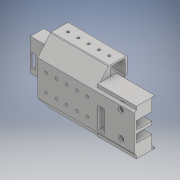
# Autodesk Inventor part: MagnetHousing_SmallGrad
Saved by Autodesk Inventor 2017 (Build 210142000, 142)
## iProperties
Created: 2017-04-05
Part Number: MagnetHousing_SmallGrad
Material: Generic
Document SubType Name: Modeling
Designer: greer_000
Density: 1 g/cm^3
Appearance: Default
Mass: 46.9919 g
Surface Area: 340.055 cm^2
Volume: 46.9919 cm^3
Author: greer_000
Autodesk Inventor part; units mm, degrees
ref_plane "YZ Plane" through (0, 0, 0) normal (1, 0, 0) x (0, 1, 0)
ref_plane "XZ Plane" through (0, 0, 0) normal (0, 1, 0) x (-1, 0, 0)
ref_plane "XY Plane" through (0, 0, 0) normal (0, 0, 1) x (1, 0, 0)
sketch "Sketch1" plane through (0, 0, 0) normal (1, 0, 0) x (0, 1, 0)
  line L0 (0, 0) -> (0, 17)
  line L1 (0, 17) -> (12.3002, 31.677)
  line L2 (13.0667, 32.0347) -> (29.3, 32.0347)
  line L3 (30.3, 31.0347) -> (30.3, 16.2862)
  line L4 (16.75, 10.8595) -> (16.75, 0)
  line L5 (29.5781, 15.3257) -> (17.4719, 11.8201)
  line L6 (0, 0) -> (0, -17)
  line L7 (0, -17) -> (12.3002, -31.677)
  line L8 (13.0667, -32.0347) -> (29.3, -32.0347)
  line L9 (30.3, -31.0347) -> (30.3, -16.2862)
  line L10 (16.75, -10.8595) -> (16.75, 0)
  line L11 (29.5781, -15.3257) -> (17.4719, -11.8201)
  arc A0 (29.3, -32.0347) -> (30.3, -31.0347) centre (29.3, -31.0347) ccw
  arc A1 (30.3, -16.2862) -> (29.5781, -15.3257) centre (29.3, -16.2862) ccw
  arc A2 (29.5781, 15.3257) -> (30.3, 16.2862) centre (29.3, 16.2862) ccw
  arc A3 (30.3, 31.0347) -> (29.3, 32.0347) centre (29.3, 31.0347) ccw
  arc A4 (13.0667, 32.0347) -> (12.3002, 31.677) centre (13.0667, 31.0347) ccw
  arc A5 (12.3002, -31.677) -> (13.0667, -32.0347) centre (13.0667, -31.0347) ccw
  line L12 (17.4719, 11.8201) -> (16.75, 11.6111)
  line L13 (16.75, 11.6111) -> (16.75, 10.8595)
  line L14 (17.4719, -11.8201) -> (16.75, -11.611)
  line L15 (16.75, -11.611) -> (16.75, -10.8595)
  point P0 (12.6, 32.0347)
  point P1 (30.3, 32.0347)
  point P2 (30.3, 15.5347)
  point P3 (12.6, -32.0347)
  point P4 (30.3, -32.0347)
  point P5 (30.3, -15.5347)
  point P6 (16.75, -11.6111)
  dimension "d1" = 17
  dimension "d3" = 17.7
  dimension "d4" = 30.3
  dimension "d5" = 16.5
  dimension "d6" = 16.75
  dimension "d7" = 11.6111
  dimension "d186" = 11.6111
  dimension "d187" = 17.7
  dimension "d188" = 30.3
  dimension "d189" = 16.5
  dimension "d191" = 15.0347
  dimension "d192" = 17
  dimension "d297" = 15.0347
  dimension "d308" = 3.9236
  dimension "d309" = 3.9236
  dimension "d325" = 1
  constraints: 32 end point, 16 point on line, 12 point on circle, 12 tangent, 6 centre point, 5 equal radius, 5 vertical, 1 horizontal
  measures "d1" distance of L0.start L0.end
  measures "d3" distance of point (12.6, 32.035) point (30.3, 32.035)
  measures "d4" horizontal distance of L0.end point (30.3, 32.035)
  measures "d5" distance of point (30.3, 32.035) point (30.3, 15.535)
  measures "d6" distance between parallel lines of L4 L0
  measures "d7" distance of L12.end L4.end
  measures "d186" distance of point (16.75, -11.611) L4.end
  measures "d187" distance of point (12.6, -32.035) point (30.3, -32.035)
  measures "d188" distance from line of L7.start L9
  measures "d189" distance of point (30.3, -32.035) point (30.3, -15.535)
  measures "d191" vertical distance of point (12.6, -32.035) L7.start
  measures "d192" distance of L0.start L7.start
  measures "d297" vertical distance of point (12.6, 32.035) L0.end
  measures "d308" vertical distance of L12.end point (30.3, 15.535)
  measures "d309" vertical distance of point (30.3, -15.535) point (16.75, -11.611)
  measures "d325" radius of A0
extrude "Extrusion1" add sketch "Sketch1" against normal blind 56.3
sketch "Sketch2" plane through (0, 0, 0) normal (1, 0, 0) x (0, 0, -1)
  line L0 (-29.4847, 28.55) -> (-16.5847, 28.55)
  line L1 (-15.5847, 27.55) -> (-15.5847, 14.325)
  line L2 (-30.4847, 15.325) -> (-30.4847, 27.55)
  line L3 (-32.0347, 13.0667) -> (-32.0347, 29.3) projected
  line L4 (17, 0) -> (-17, 0) projected
  line L5 (-11.6111, 16.75) -> (11.6111, 16.75) projected
  line L6 (0, 16.75) -> (0, 3.3802)
  line L7 (29.4847, 28.55) -> (16.5847, 28.55)
  line L8 (15.5847, 27.55) -> (15.5847, 14.325)
  line L9 (15.5847, 14.325) -> (29.4847, 14.325)
  line L10 (30.4847, 15.325) -> (30.4847, 27.55)
  line L11 (-14.4375, 15.9) -> (14.438, 15.9)
  line L12 (14.438, 15.9) -> (14.438, 1.75)
  line L13 (14.438, 1.75) -> (-14.4375, 1.75)
  line L14 (-14.4375, 1.75) -> (-14.4375, 15.9)
  line L15 (-31.0347, 30.3) -> (-16.2862, 30.3) projected
  arc A0 (-15.5847, 27.55) -> (-16.5847, 28.55) centre (-16.5847, 27.55) ccw
  arc A1 (-29.4847, 28.55) -> (-30.4847, 27.55) centre (-29.4847, 27.55) ccw
  arc A2 (16.5847, 28.55) -> (15.5847, 27.55) centre (16.5847, 27.55) ccw
  arc A3 (30.4847, 27.55) -> (29.4847, 28.55) centre (29.4847, 27.55) ccw
  arc A4 (29.4847, 14.325) -> (30.4847, 15.325) centre (29.4847, 15.325) ccw
  line L16 (-15.5847, 14.325) -> (-29.4847, 14.325)
  line L17 (-30.4847, 15.325) -> (-30.4847, 15.325)
  arc A5 (-30.4847, 15.325) -> (-29.4847, 14.325) centre (-29.4847, 15.325) ccw
  line L18 (-16.0847, 14.325) -> (-28.7847, 14.325) construction
  line L19 (-28.7847, 14.325) -> (-28.7847, 27.025) construction
  line L20 (-28.7847, 27.025) -> (-16.0847, 27.025) construction
  line L21 (-16.0847, 27.025) -> (-16.0847, 14.325) construction
  line L22 (-28.7847, 20.675) -> (-4.4905, 20.675) construction
  line L23 (-12.9889, 15.4) -> (6.9303, 15.4) construction
  line L24 (16.0847, 14.325) -> (28.7847, 14.325) construction
  line L25 (28.7847, 14.325) -> (28.7847, 27.025) construction
  line L26 (28.7847, 27.025) -> (16.0847, 27.025) construction
  line L27 (16.0847, 27.025) -> (16.0847, 14.325) construction
  line L28 (16.0847, 20.675) -> (4.3729, 20.675) construction
  line L29 (-22.4347, 27.025) -> (-22.4347, 13.0667) construction
  point P0 (0, 0)
  point P1 (-30.4847, 28.55)
  point P2 (-15.5847, 28.55)
  point P3 (-30.4847, 14.325)
  point P4 (-32.0347, 12.6)
  point P5 (-32.0347, 30.3)
  point P6 (30.4847, 28.55)
  point P7 (15.5847, 28.55)
  point P8 (30.4847, 14.325)
  point P9 (-15.5347, 30.3)
  point P10 (-10.8595, 16.75)
  point P11 (10.8595, 16.75)
  dimension "d11" = 1.55
  dimension "d15" = 1.75
  dimension "d16" = 14.4375
  dimension "d17" = 14.438
  dimension "d295" = 1.75
  dimension "d296" = 0.85
  dimension "d316" = 15.5847
  dimension "d320" = 1
  dimension "d324" = 1
  dimension "d397" = 12.225
  dimension "d399" = 13.225
  dimension "d400" = 12.225
  dimension "d406" = 1
  dimension "d407" = 12.7
  dimension "d408" = 12.7
  dimension "d409" = 0.5
  dimension "d410" = 0.5
  dimension "d411" = 12.7
  dimension "d412" = 12.7
  dimension "d413" = 0.5
  constraints: 52 end point, 16 point on line, 12 point on circle, 12 tangent, 6 centre point, 6 horizontal, 6 parallel, 4 midpoint, 4 perpendicular, 4 symmetric about line, 3 equal radius, 1 vertical
  measures "d11" distance between parallel lines of L2 L3
  measures "d15" distance between parallel lines of L13 L4
  measures "d16" distance between parallel lines of L6 L14
  measures "d17" distance between parallel lines of L6 L12
  measures "d295" distance between parallel lines of L15 L0
  measures "d296" distance between parallel lines of L5 L11
  measures "d316" distance between parallel lines of L6 L1
  measures "d320" radius of A0
  measures "d324" radius of A2
  measures "d397" distance of L2.start L2.end
  measures "d399" distance of L1.start L1.end
  measures "d400" distance of L10.start L10.end
  measures "d406" radius of A5
  measures "d407" distance of L19.end L20.end
  measures "d408" distance of L18.end L19.end
  measures "d409" distance between parallel lines of L1 L21
  measures "d410" distance between parallel lines of L11 L23
  measures "d411" distance of L26.end L25.end
  measures "d412" distance of L25.end L24.end
  measures "d413" distance between parallel lines of L8 L27
extrude "Extrusion2" cut sketch "Sketch2" against normal up to next
sketch "Sketch35" plane through (0, 0, 0) normal (1, 0, 0) x (0, 0, -1)
  line L0 (-11.6111, 16.75) -> (11.6111, 16.75) projected
  line L1 (-11.6111, 16.75) -> (-15.7347, 16.75)
  line L2 (-15.7347, 16.75) -> (-15.7347, 15.9)
  line L3 (-15.7347, 15.9) -> (15.5847, 15.9)
  line L4 (15.5847, 14.325) -> (15.5847, 27.55) projected
  line L5 (15.5847, 15.9) -> (15.5847, 16.75)
  line L6 (15.5847, 16.75) -> (11.6111, 16.75)
  line L7 (-11.6111, 16.75) -> (11.6111, 16.75)
  point P0 (0, 0)
  point P1 (15.5847, 28.8)
  point P2 (-10.8595, 16.75)
  point P3 (10.8595, 16.75)
  constraints: 12 end point, 2 collinear, 2 vertical, 1 horizontal, 1 perpendicular, 1 point on line
extrude "Extrusion32" add sketch "Sketch35" along normal blind 8.062
sketch "Sketch36" plane through (-56.3, 16.75, -11.611) normal (0, 1, 0) x (1, 0, 0)
  circle A0 centre (61.362, -17.6111) radius 1.505
  circle A1 centre (61.362, -11.6111) radius 1.505
  circle A2 centre (61.362, -5.6111) radius 1.505
  line L0 (64.362, 3.9736) -> (64.362, -27.3457) projected
  point P0 (56.3, -11.6111)
  dimension "d195" = 3.01
  dimension "d196" = 3.01
  dimension "d197" = 3.01
  dimension "d198" = 3
  dimension "d200" = 3
  dimension "d201" = 0
  dimension "d202" = 3
  dimension "d203" = 6
  dimension "d204" = 6
  constraints: 3 centre point
  measures "d195" diameter of A0
  measures "d196" diameter of A1
  measures "d197" diameter of A2
  measures "d198" distance from line of L0 A0.centre
  measures "d200" distance from line of L0 A2.centre
  measures "d201" vertical distance of point (56.3, -11.611) A1.centre
  measures "d202" distance from line of A1.centre L0
  measures "d203" distance of A2.centre A1.centre
  measures "d204" distance of A0.centre A1.centre
extrude "Extrusion33" cut sketch "Sketch36" against normal blind 8.062
sketch "Sketch37" plane through (0, 14.325, -15.5847) normal (0, 0, -1) x (-1, 0, 0)
  line L0 (0, 2.425) -> (-8.062, 2.425) projected
  line L1 (0, 1.575) -> (-8.062, 1.575) projected
  line L2 (-8.062, 2.425) -> (0, 2.425)
  line L3 (0, 2.425) -> (0, 1.075)
  line L4 (0, 1.075) -> (-8.062, 1.075)
  line L5 (-8.062, 1.075) -> (-8.062, 2.425)
  point P0 (0, -14.325)
  constraints: 8 end point, 2 parallel, 1 horizontal, 1 perpendicular, 1 other
extrude "Extrusion34" add sketch "Sketch37" along normal blind 4.9105
sketch "Sketch38" plane through (0, 14.325, 15.5847) normal (0, 0, 1) x (1, 0, 0)
  line L0 (8.062, 2.425) -> (8.062, 1.575) projected
  line L1 (8.062, 2.425) -> (0, 2.425)
  line L2 (0, 2.425) -> (0, 1.575)
  line L3 (0, 1.575) -> (8.062, 1.575)
  line L4 (8.062, 1.575) -> (8.062, 2.425)
  point P0 (0, -14.325)
  constraints: 8 end point, 2 parallel, 1 horizontal, 1 perpendicular
extrude "Extrusion35" add sketch "Sketch38" along normal blind 4.9105
sketch "Sketch39" plane through (8.062, 0, 0) normal (1, 0, 0) x (0, 0, -1)
  line L0 (-15.5847, 16.75) -> (-20.4952, 16.75) projected
  line L1 (15.5847, 15.4) -> (20.4952, 15.4) projected
  line L2 (-20.4952, 16.75) -> (20.4952, 16.75)
  line L3 (20.4952, 16.75) -> (20.4952, 15.4)
  line L4 (20.4952, 15.4) -> (-20.4952, 15.4)
  line L5 (-20.4952, 15.4) -> (-20.4952, 16.75)
  point P0 (0, 0)
  point P1 (15.5847, 15.9)
  constraints: 8 end point, 2 parallel, 1 horizontal, 1 perpendicular, 1 other
extrude "Extrusion36" add sketch "Sketch39" along normal blind 29.6
sketch "Sketch40" plane through (-56.3, 16.75, -11.611) normal (0, 1, 0) x (1, 0, 0)
  line L0 (85.241, 1.9681) -> (91.351, 1.9681)
  line L1 (91.351, 1.9681) -> (91.351, 7.4181)
  line L2 (91.351, 7.4181) -> (85.241, 7.4181)
  line L3 (85.241, 7.4181) -> (85.241, 1.9681)
  line L4 (56.3, 8.8841) -> (93.962, 8.8841) projected
  line L5 (93.962, -32.1062) -> (93.962, 8.8841) projected
  circle A0 centre (80.723, -1.2209) radius 6.25
  point P0 (56.3, -11.6111)
  dimension "d213" = 6.11
  dimension "d214" = 5.45
  dimension "d215" = 1.466
  dimension "d216" = 2.611
  dimension "d217" = 12.5
  dimension "d218" = 10.105
  dimension "d219" = 13.239
  constraints: 8 end point, 2 parallel, 1 centre point, 1 horizontal, 1 perpendicular
  measures "d213" distance of L1.end L2.end
  measures "d214" distance of L2.end L0.start
  measures "d215" distance between parallel lines of L4 L2
  measures "d216" distance between parallel lines of L5 L1
  measures "d217" diameter of A0
  measures "d218" distance from line of L4 A0.centre
  measures "d219" distance from line of L5 A0.centre
extrude "Extrusion37" cut sketch "Sketch40" against normal blind 29.6
sketch "Sketch41" plane through (-56.3, 16.75, -11.611) normal (0, 1, 0) x (1, 0, 0)
  line L0 (84.662, -21.7659) -> (93.962, -21.7659)
  line L1 (93.962, -21.7659) -> (93.962, -13.7659)
  line L2 (93.962, -13.7659) -> (84.662, -13.7659)
  line L3 (84.662, -13.7659) -> (84.662, -21.7659)
  line L4 (84.662, -10.8659) -> (93.962, -10.8659)
  line L5 (93.962, -10.8659) -> (93.962, -2.8659)
  line L6 (93.962, -2.8659) -> (84.662, -2.8659)
  line L7 (84.662, -2.8659) -> (84.662, -10.8659)
  line L8 (56.3, 8.8841) -> (93.962, 8.8841) projected
  line L9 (93.962, 8.8841) -> (93.962, -32.1062) projected
  point P0 (56.3, -11.6111)
  dimension "d222" = 9.3
  dimension "d223" = 8
  dimension "d224" = 8
  dimension "d225" = 11.75
  dimension "d227" = 22.65
  dimension "d243" = 0
  constraints: 16 end point, 4 parallel, 2 horizontal, 2 perpendicular, 2 point on line
  measures "d222" distance of L0.start L0.end
  measures "d223" distance of L2.end L0.start
  measures "d224" distance of L6.end L4.start
  measures "d225" distance between parallel lines of L8 L6
  measures "d227" distance between parallel lines of L8 L2
  measures "d243" distance between parallel lines of L9 L1
extrude "Extrusion38" cut sketch "Sketch41" against normal blind 29.6
sketch "Sketch42" plane through (-56.3, 16.75, -11.611) normal (0, 1, 0) x (1, 0, 0)
  circle A0 centre (80.604, -25.0282) radius 6.25
  line L0 (56.3, -32.1062) -> (93.962, -32.1062) projected
  line L1 (93.962, 8.8841) -> (93.962, -32.1062) projected
  line L2 (75.873, -15.0931) -> (83.551, -15.0931)
  line L3 (83.551, -15.0931) -> (83.551, -9.6387)
  line L4 (83.551, -9.6387) -> (75.873, -9.6387)
  line L5 (75.873, -9.6387) -> (75.873, -15.0931)
  line L6 (56.3, 8.8841) -> (93.962, 8.8841) projected
  point P0 (56.3, -11.6111)
  dimension "d230" = 12.5
  dimension "d231" = 7.078
  dimension "d232" = 13.358
  dimension "d237" = 18.5228
  dimension "d238" = 5.4544
  dimension "d239" = 10.411
  dimension "d240" = 7.678
  constraints: 8 end point, 2 parallel, 1 centre point, 1 horizontal, 1 perpendicular
  measures "d230" diameter of A0
  measures "d231" distance from line of L0 A0.centre
  measures "d232" distance from line of L1 A0.centre
  measures "d237" distance between parallel lines of L6 L4
  measures "d238" distance of L4.end L2.start
  measures "d239" distance between parallel lines of L1 L3
  measures "d240" distance of L2.start L2.end
extrude "Extrusion39" cut sketch "Sketch42" against normal blind 29.6
sketch "Sketch43" plane through (-56.3, 16.75, -11.611) normal (0, 1, 0) x (1, 0, 0)
  line L0 (69.359, -17.8987) -> (73.747, -17.8987)
  line L1 (73.747, -17.8987) -> (73.747, -8.4307)
  line L2 (73.747, -8.4307) -> (69.359, -8.4307)
  line L3 (69.359, -8.4307) -> (69.359, -17.8987)
  line L4 (93.962, -21.7659) -> (93.962, -32.1062) projected
  line L5 (56.3, 8.8841) -> (93.962, 8.8841) projected
  point P0 (56.3, -11.6111)
  dimension "d244" = 9.468
  dimension "d245" = 4.388
  dimension "d246" = 20.215
  dimension "d247" = 17.3148
  constraints: 8 end point, 2 parallel, 1 horizontal, 1 perpendicular
  measures "d244" distance of L2.end L0.start
  measures "d245" distance of L1.end L2.end
  measures "d246" distance between parallel lines of L4 L1
  measures "d247" distance between parallel lines of L5 L2
extrude "Extrusion40" cut sketch "Sketch43" against normal blind 29.6
sketch "Sketch44" plane through (0, 0, 0) normal (1, 0, 0) x (0, 0, -1)
  line L0 (-14.4375, 1.75) -> (14.438, 1.75) projected
  line L1 (17, 0) -> (-17, 0) projected
  line L2 (-17, 0) -> (17, 0)
  line L3 (14.438, 1.75) -> (-14.4375, 1.75)
  line L4 (31.677, 12.3002) -> (17, 0) projected
  line L5 (14.438, 1.75) -> (19.0882, 1.75)
  line L6 (17, 0) -> (19.0882, 1.75)
  line L7 (-14.4375, 1.75) -> (-19.0882, 1.75)
  line L8 (-17, 0) -> (-31.677, 12.3002) projected
  line L9 (-19.0882, 1.75) -> (-17, 0)
  point P0 (0, 0)
  point P1 (32.0347, 12.6)
  dimension "d336" = 4.6506
  constraints: 12 end point, 3 horizontal, 2 collinear, 1 point on line
  measures "d336" distance of L0.start L7.end
extrude "Extrusion41" add sketch "Sketch44" along normal blind 37.662
sketch "Sketch45" plane through (-56.3, 16.75, -11.611) normal (0, 1, 0) x (1, 0, 0)
  line L0 (93.962, -21.7659) -> (85.935, -21.7659) projected
  line L1 (93.962, -32.1062) -> (93.962, -21.7659)
  line L2 (93.962, -21.7659) -> (85.935, -21.7659)
  arc A0 (84.662, -20.2748) -> (85.935, -21.7659) centre (80.604, -25.0282) ccw projected
  arc A1 (84.662, -29.7817) -> (85.935, -21.7659) centre (80.604, -25.0282) ccw
  line L3 (84.662, -29.7817) -> (84.662, -32.1062)
  line L4 (84.662, -32.1062) -> (93.962, -32.1062)
  line L5 (84.662, -6.0734) -> (84.662, -10.8659) projected
  line L6 (84.662, -13.7662) -> (84.662, -10.8659)
  line L7 (84.662, -10.8659) -> (93.962, -10.8659) projected
  line L8 (84.662, -10.8659) -> (93.962, -10.8659)
  line L9 (93.962, -10.8659) -> (93.962, -13.7662)
  line L10 (93.962, -28.6111) -> (93.962, 5.3889) projected
  line L11 (84.662, -13.7662) -> (93.962, -13.7662)
  line L12 (93.962, -2.8659) -> (86.7526, -2.8659) projected
  line L13 (93.962, -2.8659) -> (86.7526, -2.8659)
  arc A2 (86.7526, -2.8659) -> (86.0982, 1.9681) centre (80.723, -1.2209) ccw projected
  arc A3 (86.7526, -2.8659) -> (86.0982, 1.9681) centre (80.9931, -1.1843) ccw
  line L14 (86.0982, 1.9681) -> (91.351, 1.9681) projected
  line L15 (86.0982, 1.9681) -> (91.351, 1.9681)
  line L16 (91.351, 1.9681) -> (91.351, 7.4181)
  line L17 (91.351, 7.4181) -> (85.241, 7.4181) projected
  line L18 (91.351, 7.4181) -> (85.241, 7.4181)
  line L19 (85.241, 7.4181) -> (85.241, 8.8841)
  line L20 (56.3, 8.8841) -> (93.962, 8.8841) projected
  line L21 (93.962, 8.8841) -> (85.241, 8.8841)
  line L22 (93.962, 8.8841) -> (93.962, -2.8659)
  line L23 (56.3, -32.1062) -> (93.962, -32.1062) projected
  point P0 (56.3, -11.6111)
  point P1 (93.962, 8.0737)
  dimension "d338" = 0
  constraints: 30 end point, 5 collinear, 5 point on circle, 4 perpendicular, 3 point on line, 3 vertical, 2 centre point, 1 concentric, 1 horizontal
  measures "d338" distance between parallel lines of L23 L4
extrude "Extrusion42" add sketch "Sketch45" against normal up to surface (15 mm away) contours L1 L4 L3 A0 L0 | L6 L7 L9 L11 | L12 A3 L14 L16 L17 L19 L20 L22 L10
sketch "Sketch46" plane through (-56.3, 16.75, -11.611) normal (0, 1, 0) x (1, 0, 0)
  line L0 (56.3, -27.1957) -> (56.3, -41.0957) projected
  line L1 (84.662, -30.6992) -> (84.662, -29.7817) projected
  line L2 (56.3, -32.3892) -> (84.662, -32.3892)
  line L3 (84.662, -32.3892) -> (84.662, -29.7817)
  arc A0 (84.662, -29.7817) -> (85.935, -21.7659) centre (80.604, -25.0282) ccw projected
  arc A1 (84.662, -20.2748) -> (84.662, -29.7817) centre (80.604, -25.0282) ccw
  line L4 (84.662, -10.8659) -> (84.662, -6.0734) projected
  line L5 (84.662, -20.2748) -> (84.662, -6.0734)
  line L6 (85.241, 7.4181) -> (85.241, 3.0977) projected
  arc A2 (85.241, 3.0977) -> (84.662, -6.0734) centre (81.1316, -1.2467) ccw
  line L7 (85.241, 3.0977) -> (85.241, 7.4181)
  line L8 (85.241, 7.4181) -> (85.241, 8.8841)
  line L9 (56.3, 8.8841) -> (93.962, 8.8841) projected
  line L10 (56.3, 8.8841) -> (85.241, 8.8841)
  line L11 (56.3, 8.8841) -> (56.3, -32.3892)
  circle A3 centre (61.362, -17.6111) radius 1.505 projected
  circle A4 centre (61.362, -17.6111) radius 1.505
  circle A5 centre (61.362, -11.6111) radius 1.505 projected
  circle A6 centre (61.362, -11.6111) radius 1.505
  circle A7 centre (61.362, -5.6111) radius 1.505 projected
  circle A8 centre (61.362, -5.6111) radius 1.505
  line L12 (69.359, -8.4307) -> (69.359, -17.8987) projected
  line L13 (69.359, -17.8987) -> (73.747, -17.8987)
  line L14 (73.747, -17.8987) -> (73.747, -8.4307)
  line L15 (73.747, -8.4307) -> (69.359, -8.4307)
  line L16 (69.359, -8.4307) -> (69.359, -17.8987)
  line L17 (75.873, -9.6387) -> (83.551, -9.6387) projected
  line L18 (75.873, -15.0931) -> (75.873, -9.6387) projected
  line L19 (75.873, -15.0931) -> (83.551, -15.0931)
  line L20 (83.551, -15.0931) -> (83.551, -9.6387)
  line L21 (83.551, -9.6387) -> (75.873, -9.6387)
  line L22 (75.873, -9.6387) -> (75.873, -15.0931)
  point P0 (56.3, -11.6111)
  point P1 (56.3, -42.0957)
  constraints: 30 end point, 5 centre point, 5 collinear, 4 parallel, 4 point on circle, 3 coincident, 3 perpendicular, 3 point on line, 2 horizontal, 1 concentric
extrude "Extrusion43" add sketch "Sketch46" against normal up to surface (15 mm away)
sketch "Sketch47" plane through (0, 1.75, 19.0882) normal (0, 1, 0) x (1, 0, 0)
  line L0 (2.0246, 12.9654) -> (8.4358, 12.9654)
  line L1 (8.4358, 12.9654) -> (8.4358, 34.055)
  line L2 (8.4358, 34.055) -> (2.0246, 34.055)
  line L3 (2.0246, 34.055) -> (2.0246, 12.9654)
  point P0 (0, 19.0882)
  constraints: 8 end point, 2 parallel, 1 horizontal, 1 perpendicular
extrude "Extrusion44" cut sketch "Sketch47" against normal blind 37.662
sketch "Sketch48" plane through (-56.3, 0, 0) normal (-1, 0, 0) x (0, 0, 1)
  line L0 (-14.438, 15.9) -> (-15.5847, 15.9)
  line L1 (-15.5847, 16.75) -> (-15.5847, 27.55) projected
  line L2 (-15.5847, 15.9) -> (-15.5847, 28.8)
  line L3 (-14.438, 15.9) -> (15.5847, 15.9)
  line L4 (15.5847, 15.9) -> (15.5847, 28.8)
  line L5 (15.5847, 28.8) -> (14.9194, 28.8)
  line L6 (14.9194, 28.8) -> (11.6111, 16.75)
  line L7 (-15.5847, 28.8) -> (-14.9194, 28.8)
  line L8 (-14.9194, 28.8) -> (-11.6111, 16.75)
  line L9 (-11.6111, 16.75) -> (11.6111, 16.75)
  line L10 (10.1548, 16.75) -> (-0.7452, 16.75) projected
  point P0 (0, 0)
  point P1 (20.6452, 16.75)
  constraints: 18 end point, 4 horizontal, 2 collinear, 1 vertical
extrude "Extrusion46" add sketch "Sketch48" along normal blind 22.938
sketch "Sketch49" plane through (0, 16.75, -15.5847) normal (0, 1, 0) x (1, 0, 0)
  circle A0 centre (-59.238, -15.5844) radius 1.5
  circle A1 centre (5.062, -15.5847) radius 1.505 projected
  circle A2 centre (-59.238, -21.5844) radius 1.5
  circle A3 centre (-59.238, -9.5844) radius 1.5
  point P0 (0, -15.5847)
  dimension "d262" = 3
  dimension "d263" = 64.3
  dimension "d264" = 3
  dimension "d265" = 3
  dimension "d266" = 6
  dimension "d267" = 6
  constraints: 3 centre point
  measures "d262" diameter of A0
  measures "d263" distance of A1.centre A0.centre
  measures "d264" diameter of A2
  measures "d265" diameter of A3
  measures "d266" distance of A2.centre A0.centre
  measures "d267" distance of A0.centre A3.centre
extrude "Extrusion47" cut sketch "Sketch49" against normal blind 22.938 contours A0 | A2 | A3
sketch "Sketch50" plane through (0, 1.75, 19.0882) normal (0, -1, 0) x (1, 0, 0)
  line L0 (8.4358, -12.9654) -> (2.0246, -12.9654)
  line L1 (2.0246, -12.9654) -> (2.0246, -34.055)
  line L2 (2.0246, -34.055) -> (8.4358, -34.055)
  line L3 (8.4358, -34.055) -> (8.4358, -12.9654)
  point P0 (0, -19.0882)
  constraints: 8 end point, 2 parallel, 1 horizontal, 1 perpendicular
extrude "Extrusion48" cut sketch "Sketch50" against normal blind 12
sketch "Sketch51" plane through (0, 16.75, -15.5847) normal (0, 1, 0) x (1, 0, 0)
  line L0 (28.362, -36.0799) -> (37.662, -36.0799) projected
  line L1 (0, 4.9105) -> (37.662, 4.9105) projected
  line L2 (39.1986, -36.0799) -> (38.4986, -36.0799)
  line L3 (38.4986, -36.0799) -> (38.4986, 4.9105)
  line L4 (38.4986, 4.9105) -> (39.1986, 4.9105)
  line L5 (39.1986, 4.9105) -> (39.1986, -36.0799)
  point P0 (0, -15.5847)
  point P1 (0, -36.3799)
  point P2 (37.662, -36.3799)
  dimension "d272" = 0.7
  constraints: 8 end point, 2 parallel, 1 horizontal, 1 perpendicular, 1 point on line, 2 other
  measures "d272" distance of L3.end L4.end
extrude "Extrusion49" cut sketch "Sketch51" against normal blind 14.3
sketch "Sketch52" plane through (29.635, 1.75, 10.1548) normal (0, 1, 0) x (1, 0, 0)
  arc A0 (-1.273, 1.4911) -> (0, 0) centre (-5.331, -3.2624) ccw projected
  circle A1 centre (-5.331, -3.2624) radius 2.5
  arc A2 (1.0133, 18.9) -> (0.3588, 23.734) centre (-4.7463, 20.5816) ccw projected
  circle A3 centre (-4.7463, 20.5816) radius 2.5
  point P0 (-29.635, 10.1548)
  point P1 (-1.0774, -8.3158)
  dimension "d275" = 5
  dimension "d276" = 5
  constraints: 2 centre point, 2 coincident, 1 other
  measures "d275" diameter of A1
  measures "d276" diameter of A3
extrude "Extrusion50" cut sketch "Sketch52" against normal up to next
sketch "Sketch57" plane through (28.941, 16.75, -19.0292) normal (0, 1, 0) x (1, 0, 0)
  line L0 (-103.279, -21.9181) -> (-107.219, -21.9181)
  line L1 (-107.219, -21.9181) -> (-107.219, -8.4581)
  line L2 (-107.219, -8.4581) -> (-103.279, -8.4581)
  line L3 (-103.279, -8.4581) -> (-103.279, -21.9181)
  circle A0 centre (-88.179, -19.0289) radius 1.5 projected
  line L4 (-28.941, -7.4181) -> (-108.179, -7.4181) projected
  point P0 (-28.941, -19.0292)
  dimension "d288" = 15.1
  dimension "d289" = 3.94
  dimension "d291" = 1.04
  dimension "d292" = 14.5
  constraints: 8 end point, 2 parallel, 1 horizontal, 1 perpendicular
  measures "d288" distance from line of A0.centre L3
  measures "d289" distance of L0.start L0.end
  measures "d291" distance between parallel lines of L4 L2
  measures "d292" distance between parallel lines of L4 L0
extrude "Extrusion54" cut sketch "Sketch57" against normal blind 18 contours L0 L1 L2 L3
sketch "Sketch60" plane through (0, 14.325, 20.4952) normal (0, 0, 1) x (1, 0, 0)
  line L0 (0, 2.425) -> (37.662, 2.425) projected
  line L1 (37.662, -12.575) -> (0, -12.575) projected
  line L2 (37.662, 2.425) -> (28.362, 2.425)
  line L3 (28.362, 2.425) -> (28.362, -12.575)
  line L4 (28.362, -12.575) -> (37.662, -12.575)
  line L5 (37.662, -12.575) -> (37.662, 2.425)
  line L6 (28.362, 2.425) -> (28.362, -12.575) projected
  point P0 (0, -14.325)
  dimension "d339" = 0
  constraints: 8 end point, 2 parallel, 1 horizontal, 1 perpendicular, 1 point on line
  measures "d339" distance between parallel lines of L6 L3
extrude "Extrusion57" add sketch "Sketch60" along normal up to surface (0.283 mm away)
sketch "Sketch61" plane through (0, 16.75, 20.7782) normal (0, 0, 1) x (1, 0, 0)
  line L0 (37.662, 0) -> (37.662, -15) projected
  line L1 (0, -15) -> (-56.3, -15) projected
  line L2 (37.662, 0) -> (0, 0)
  line L3 (0, 0) -> (0, -15)
  line L4 (0, -15) -> (37.662, -15)
  line L5 (37.662, -15) -> (37.662, 0)
  point P0 (0, -16.75)
  constraints: 8 end point, 2 parallel, 1 horizontal, 1 perpendicular
extrude "Extrusion58" add sketch "Sketch61" along normal blind 1.5
sketch "Sketch62" plane through (0, 16.75, -15.5847) normal (0, 1, 0) x (1, 0, 0)
  line L0 (37.662, -37.8628) -> (0, -37.8628) projected
  line L1 (37.662, -25.7395) -> (37.662, -37.8628) projected
  line L2 (0, -37.8628) -> (37.662, -37.8628)
  line L3 (37.662, -37.8628) -> (37.662, -37.1128)
  line L4 (37.662, -37.1128) -> (0, -37.1128)
  line L5 (0, -37.1128) -> (0, -37.8628)
  point P0 (0, -15.5847)
  dimension "d344" = 0.75
  constraints: 8 end point, 2 parallel, 1 horizontal, 1 perpendicular, 1 point on line
  measures "d344" distance of L3.end L2.end
extrude "Extrusion59" add sketch "Sketch62" along normal blind 3
sketch "Sketch63" plane through (0, 14.325, -20.4952) normal (0, 0, -1) x (-1, 0, 0)
  line L0 (-37.662, 2.425) -> (-37.662, -12.575) projected
  line L1 (0, -12.575) -> (-37.662, -12.575) projected
  line L2 (-37.662, 2.425) -> (0, 2.425)
  line L3 (0, 2.425) -> (0, -12.575)
  line L4 (0, -12.575) -> (-37.662, -12.575)
  line L5 (-37.662, -12.575) -> (-37.662, 2.425)
  point P0 (0, -14.325)
  constraints: 8 end point, 2 parallel, 1 horizontal, 1 perpendicular
extrude "Extrusion60" add sketch "Sketch63" along normal blind 1.5
sketch "Sketch64" plane through (28.941, 16.75, -19.0292) normal (0, 1, 0) x (1, 0, 0)
  line L0 (-28.941, 2.966) -> (8.721, 2.966) projected
  line L1 (8.721, 0.059) -> (8.721, 2.966) projected
  line L2 (-28.941, 2.966) -> (8.721, 2.966)
  line L3 (8.721, 2.966) -> (8.721, 2.216)
  line L4 (8.721, 2.216) -> (-28.941, 2.216)
  line L5 (-28.941, 2.216) -> (-28.941, 2.966)
  point P0 (-28.941, -19.0292)
  dimension "d349" = 0.75
  constraints: 8 end point, 2 parallel, 1 horizontal, 1 perpendicular, 1 point on line
  measures "d349" distance of L2.end L3.end
extrude "Extrusion61" add sketch "Sketch64" along normal blind 3
sketch "Sketch65" plane through (0, 30.3, -16.2862) normal (0, 1, 0) x (1, 0, 0)
  circle A0 centre (-48.15, 7.3745) radius 1.2167
  line L0 (0, 14.7485) -> (-56.3, 14.7485) projected
  line L1 (0, 0) -> (-56.3, 0) projected
  line L2 (-56.3, 0) -> (-56.3, 14.7485) projected
  circle A1 centre (-38.15, 7.4085) radius 1.2167
  circle A2 centre (-28.15, 7.4085) radius 1.2165
  circle A3 centre (-18.15, 7.4085) radius 1.2166
  circle A4 centre (-8.15, 7.3742) radius 1.2166
  line L3 (0, 0) -> (0, 14.7485) projected
  line L4 (0, -16.2862) -> (-83.4131, -16.2862) construction
  circle A5 centre (-48.15, -39.9469) radius 1.2167
  circle A6 centre (-38.15, -39.9809) radius 1.2167
  circle A7 centre (-28.15, -39.9809) radius 1.2165
  circle A8 centre (-18.15, -39.9809) radius 1.2166
  circle A9 centre (-8.15, -39.9466) radius 1.2166
  dimension "d353" = 2.4333
  dimension "d354" = 7.374
  dimension "d355" = 7.3745
  dimension "d356" = 8.15
  dimension "d357" = 2.4333
  dimension "d359" = 7.34
  dimension "d360" = 2.433
  dimension "d361" = 10
  dimension "d362" = 7.34
  dimension "d363" = 2.4332
  dimension "d364" = 10
  dimension "d365" = 7.34
  dimension "d366" = 2.4332
  dimension "d367" = 10
  dimension "d368" = 8.15
  dimension "d369" = 10
  constraints: 10 centre point, 5 symmetric about line, 2 end point, 1 horizontal, 5 other
  measures "d353" diameter of A0
  measures "d354" distance from line of L0 A0.centre
  measures "d355" distance from line of L1 A0.centre
  measures "d356" distance from line of A0.centre L2
  measures "d357" diameter of A1
  measures "d359" distance from line of L0 A1.centre
  measures "d360" diameter of A2
  measures "d361" distance of A1.centre A2.centre
  measures "d362" distance from line of L0 A2.centre
  measures "d363" diameter of A3
  measures "d364" distance of A3.centre A2.centre
  measures "d365" distance from line of L0 A3.centre
  measures "d366" diameter of A4
  measures "d367" horizontal distance of A3.centre A4.centre
  measures "d368" distance from line of L3 A4.centre
  measures "d369" horizontal distance of A1.centre A0.centre
extrude "Extrusion62" cut sketch "Sketch65" against normal up to next contours A0 | A1 | A2 | A3 | A4 | A5 | A6 | A7 | A8 | A9
sketch "Sketch66" plane through (0, 13.0667, -32.0347) normal (0, 0, -1) x (-1, 0, 0)
  circle A0 centre (48.15, 8.1083) radius 1.2167
  line L0 (0, 16.2333) -> (56.3, 16.2333) projected
  circle A1 centre (38.15, 8.1083) radius 1.2166
  circle A2 centre (28.15, 8.1083) radius 1.2166
  circle A3 centre (18.15, 8.1083) radius 1.2166
  circle A4 centre (8.15, 8.1083) radius 1.2166
  line L1 (56.3, 16.2333) -> (56.3, 0) projected
  line L2 (0, 16.2333) -> (0, 0) projected
  point P0 (0, -13.0667)
  dimension "d372" = 2.4333
  dimension "d374" = 8.125
  dimension "d375" = 2.4332
  dimension "d376" = 2.4332
  dimension "d377" = 2.4332
  dimension "d378" = 2.4332
  dimension "d379" = 10
  dimension "d380" = 8.125
  dimension "d381" = 10
  dimension "d382" = 8.125
  dimension "d383" = 10
  dimension "d384" = 8.125
  dimension "d385" = 10
  dimension "d386" = 8.125
  dimension "d387" = 8.15
  dimension "d388" = 8.15
  constraints: 5 centre point
  measures "d372" diameter of A0
  measures "d374" distance from line of L0 A0.centre
  measures "d375" diameter of A1
  measures "d376" diameter of A2
  measures "d377" diameter of A3
  measures "d378" diameter of A4
  measures "d379" distance of A0.centre A1.centre
  measures "d380" distance from line of L0 A1.centre
  measures "d381" distance of A1.centre A2.centre
  measures "d382" distance from line of L0 A2.centre
  measures "d383" distance of A2.centre A3.centre
  measures "d384" distance from line of L0 A3.centre
  measures "d385" distance of A3.centre A4.centre
  measures "d386" distance from line of L0 A4.centre
  measures "d387" distance from line of L1 A0.centre
  measures "d388" distance from line of L2 A4.centre
extrude "Extrusion63" cut sketch "Sketch66" against normal up to next
sketch "Sketch67" plane through (0, 13.0667, 32.0347) normal (0, 0, 1) x (1, 0, 0)
  circle A0 centre (-48.15, 8.1083) radius 1.2166
  line L0 (-56.3, 0) -> (-56.3, 16.2333) projected
  line L1 (0, 16.2333) -> (-56.3, 16.2333) projected
  circle A1 centre (-38.15, 8.1083) radius 1.2166 projected
  circle A2 centre (-38.15, 8.1083) radius 1.2166
  circle A3 centre (-28.15, 8.1083) radius 1.2166 projected
  circle A4 centre (-28.15, 8.1083) radius 1.2166
  circle A5 centre (-18.15, 8.1083) radius 1.2166 projected
  circle A6 centre (-18.15, 8.1083) radius 1.2166
  circle A7 centre (-8.15, 8.1083) radius 1.2166 projected
  circle A8 centre (-8.15, 8.1083) radius 1.2166
  point P0 (0, -13.0667)
  dimension "d391" = 2.4332
  dimension "d392" = 8.15
  dimension "d393" = 8.125
  dimension "d394" = 10
  constraints: 5 centre point, 4 coincident
  measures "d391" diameter of A0
  measures "d392" distance from line of L0 A0.centre
  measures "d393" distance from line of L1 A0.centre
  measures "d394" distance of A0.centre A2.centre
extrude "Extrusion64" cut sketch "Sketch67" against normal up to next
sketch "Sketch68" plane through (-56.3, 0, -17) normal (0, -1, 0) x (1, 0, 0)
  circle A0 centre (8.15, 8.5) radius 1.2166
  line L0 (0, 0) -> (0, 34) projected
  line L1 (93.962, 34) -> (0, 34) projected
  line L2 (93.962, 0) -> (0, 0) projected
  circle A1 centre (18.15, 8.5) radius 1.2166
  circle A2 centre (28.15, 8.5) radius 1.2166
  circle A3 centre (38.15, 8.5) radius 1.2166
  circle A4 centre (48.15, 8.5) radius 1.2166
  circle A5 centre (8.15, 25.5) radius 1.2166
  circle A6 centre (18.15, 25.5) radius 1.2166
  circle A7 centre (28.15, 25.5) radius 1.2166
  circle A8 centre (38.15, 25.5) radius 1.2166
  circle A9 centre (48.15, 25.5) radius 1.2166
  point P0 (56.3, 17)
  dimension "d414" = 2.4332
  dimension "d415" = 8.15
  dimension "d416" = 34
  dimension "d417" = 8.5
  dimension "d420" = 10
  dimension "d423" = 17
  constraints: 10 centre point, 1 horizontal, 1 vertical, 18 other
  measures "d414" diameter of A0
  measures "d415" distance from line of L0 A0.centre
  measures "d416" distance between parallel lines of L1 L2
  measures "d417" distance from line of L2 A0.centre
  measures "d420" distance of A0.centre A1.centre
  measures "d423" distance of A0.centre A5.centre
extrude "Extrusion65" cut sketch "Sketch68" against normal up to next
body "Solid1"
